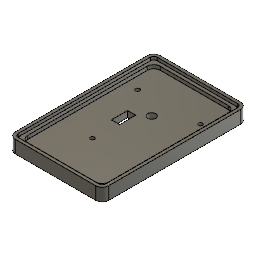
newboxtop v5 (Autodesk Fusion 360 design; units mm, degrees)
Autodesk Fusion 360 part; units mm, degrees
sketch "Sketch1" plane through (0, 0, 0) normal (0, 1, 0) x (1, 0, 0)
  line L0 (36.83, 57.15) -> (-36.83, 57.15)
  line L1 (-36.83, 57.15) -> (-36.83, -57.15)
  line L2 (-36.83, -57.15) -> (36.83, -57.15)
  line L3 (36.83, -57.15) -> (36.83, 57.15)
  line L4 (36.83, 57.15) -> (-36.83, -57.15) construction
  line L5 (-36.83, 57.15) -> (36.83, -57.15) construction
  dimension "d1" = 73.66
  dimension "d2" = 114.3
extrude "Extrude1" add sketch "Sketch1" along normal blind 10.16
shell "Shell1" thickness 4.953 removed faces 1 at (12.2767, 10.16, 19.05)
sketch "Sketch2" plane through (0, 4.953, 0) normal (0, 1, 0) x (-1, 0, 0)
  line L0 (-31.877, 52.197) -> (-31.877, -52.197)
  line L1 (-31.877, -52.197) -> (31.877, -52.197)
  line L2 (31.877, -52.197) -> (31.877, 52.197)
  line L3 (31.877, 52.197) -> (-31.877, 52.197)
  circle A0 centre (-25.8572, -31.2674) radius 1.6002
  circle A1 centre (22.4028, -29.9974) radius 1.6002
  circle A2 centre (7.1628, 20.8026) radius 1.6002
  dimension "d6" = 3.2004
  dimension "d7" = 3.2004
  dimension "d8" = 3.2004
  dimension "d9" = 6.0198
  dimension "d10" = 20.9296
  dimension "d11" = 48.26
  dimension "d12" = 22.1996
  dimension "d13" = 33.02
  dimension "d14" = 52.07
  measures "d6" diameter of A0
  measures "d7" diameter of A1
  measures "d8" diameter of A2
  measures "d13" distance of origin
  measures "d14" distance of origin
extrude "Extrude2" cut sketch "Sketch2" against normal through all contours A0 | A1 | A2
sketch "Sketch3" plane through (0, 4.953, 0) normal (0, 1, 0) x (-1, 0, 0)
  circle A0 centre (22.4028, -29.9974) radius 1.6002
  circle A1 centre (-25.8572, -31.2674) radius 1.6002
  circle A2 centre (7.1628, 20.8026) radius 1.6002
  line L0 (-31.877, 52.197) -> (-31.877, -52.197)
  line L1 (-31.877, -52.197) -> (31.877, -52.197)
  line L2 (31.877, -52.197) -> (31.877, 52.197)
  line L3 (31.877, 52.197) -> (-31.877, 52.197)
  line L4 (5.842, 0.8128) -> (12.192, 0.8128)
  line L5 (12.192, 0.8128) -> (12.192, -11.8872)
  line L6 (12.192, -11.8872) -> (5.842, -11.8872)
  line L7 (5.842, -11.8872) -> (5.842, 0.8128)
  line L8 (5.842, 0.8128) -> (12.192, -11.8872) construction
  line L9 (12.192, 0.8128) -> (5.842, -11.8872) construction
  dimension "d16" = 6.35
  dimension "d17" = 12.7
  dimension "d18" = 22.86
  dimension "d19" = 46.6598
extrude "Extrude3" cut sketch "Sketch3" against normal through all contours L4 L5 L6 L7
fillet "Fillet1" radius 5.08 8 edges at (-36.83, 5.08, 57.15) (36.83, 5.08, 57.15) (36.83, 5.08, -57.15) (-36.83, 5.08, -57.15) (31.877, 7.5565, 52.197) (31.877, 7.5565, -52.197) (-31.877, 7.5565, -52.197) (-31.877, 7.5565, 52.197)
sketch "Sketch4" plane through (0, 10.16, 0) normal (0, 1, 0) x (-1, 0, 0)
  arc A0 (31.75, -57.15) -> (36.83, -52.07) centre (31.75, -52.07) ccw
  line L0 (36.83, -52.07) -> (36.83, 52.07)
  arc A1 (36.83, 52.07) -> (31.75, 57.15) centre (31.75, 52.07) ccw
  line L1 (31.75, 57.15) -> (-31.75, 57.15)
  arc A2 (-31.75, 57.15) -> (-36.83, 52.07) centre (-31.75, 52.07) ccw
  line L2 (-36.83, 52.07) -> (-36.83, -52.07)
  arc A3 (-36.83, -52.07) -> (-31.75, -57.15) centre (-31.75, -52.07) ccw
  line L3 (-31.75, -57.15) -> (31.75, -57.15)
  line L4 (-26.797, 52.197) -> (26.797, 52.197)
  arc A4 (31.877, 47.117) -> (26.797, 52.197) centre (26.797, 47.117) ccw
  line L5 (31.877, 47.117) -> (31.877, -47.117)
  arc A5 (26.797, -52.197) -> (31.877, -47.117) centre (26.797, -47.117) ccw
  line L6 (26.797, -52.197) -> (-26.797, -52.197)
  arc A6 (-31.877, -47.117) -> (-26.797, -52.197) centre (-26.797, -47.117) ccw
  line L7 (-31.877, -47.117) -> (-31.877, 47.117)
  arc A7 (-26.797, 52.197) -> (-31.877, 47.117) centre (-26.797, 47.117) ccw
  line L8 (31.75, 54.737) -> (-31.75, 54.737)
  arc A8 (-31.75, 54.737) -> (-34.417, 52.07) centre (-31.75, 52.07) ccw
  line L9 (-34.417, 52.07) -> (-34.417, -52.07)
  arc A9 (-34.417, -52.07) -> (-31.75, -54.737) centre (-31.75, -52.07) ccw
  line L10 (-31.75, -54.737) -> (31.75, -54.737)
  arc A10 (31.75, -54.737) -> (34.417, -52.07) centre (31.75, -52.07) ccw
  line L11 (34.417, -52.07) -> (34.417, 52.07)
  arc A11 (34.417, 52.07) -> (31.75, 54.737) centre (31.75, 52.07) ccw
  dimension "d22" = 2.413
extrude "Extrude4" cut sketch "Sketch4" against normal blind 2.413 contours L8 A8 L9 A9 L10 A10 L11 A11
sketch "Sketch5" plane through (0, 4.953, 0) normal (0, 1, 0) x (-1, 0, 0)
  arc A0 (31.877, 47.117) -> (26.797, 52.197) centre (26.797, 47.117) ccw
  line L0 (26.797, 52.197) -> (-26.797, 52.197)
  arc A1 (-26.797, 52.197) -> (-31.877, 47.117) centre (-26.797, 47.117) ccw
  line L1 (-31.877, 47.117) -> (-31.877, -47.117)
  arc A2 (-31.877, -47.117) -> (-26.797, -52.197) centre (-26.797, -47.117) ccw
  line L2 (-26.797, -52.197) -> (26.797, -52.197)
  arc A3 (26.797, -52.197) -> (31.877, -47.117) centre (26.797, -47.117) ccw
  line L3 (31.877, -47.117) -> (31.877, 47.117)
  line L4 (5.842, -11.8872) -> (5.842, 0.8128)
  line L5 (5.842, 0.8128) -> (12.192, 0.8128)
  line L6 (12.192, 0.8128) -> (12.192, -11.8872)
  line L7 (12.192, -11.8872) -> (5.842, -11.8872)
  circle A4 centre (22.4028, -29.9974) radius 1.6002
  circle A5 centre (-25.8572, -31.2674) radius 1.6002
  circle A6 centre (7.1628, 20.8026) radius 1.6002
  circle A7 centre (-1.016, -17.7038) radius 3.175
  dimension "d25" = 6.35
  dimension "d26" = 34.4932
  dimension "d27" = 6.858
  measures "d25" diameter of A7
  measures "d27" distance of L4
extrude "Extrude5" cut sketch "Sketch5" against normal through all contours A7
